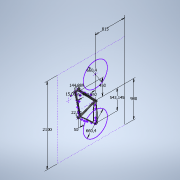
# Autodesk Inventor part: marco_bicicleta
Saved by Autodesk Inventor 2021 (Build 250183000, 183)
## iProperties
Created: 2021-06-19
Part Number: marco_bicicleta
Material: Generic
Document SubType Name: Modeling
Designer: j2seb
Density: 1 g/cm^3
Appearance: Default
Author: j2seb
Autodesk Inventor part; units mm, degrees
ref_plane "YZ Plane" through (0, 0, 0) normal (1, 0, 0) x (0, 1, 0)
ref_plane "XZ Plane" through (0, 0, 0) normal (0, 1, 0) x (-1, 0, 0)
sketch "Sketch1" plane through (0, 0, 0) normal (1, 0, 0) x (0, 1, 0)
  line L0 (-188.557163, 463.591927) -> (-1.253866, 0) construction
  line L1 (-1.253866, 0) -> (-1.253866, 463.591927) construction
  line L2 (-1.253866, 463.591927) -> (-188.557163, 463.591927) construction
  line L3 (-981.253866, 1020.526454) -> (1118.746134, 1020.526454) construction
  line L4 (1118.746134, 1020.526454) -> (1118.746134, -815) construction
  line L5 (1118.746134, -815) -> (-981.253866, -815) construction
  line L6 (-981.253866, -815) -> (-981.253866, 1020.526454) construction
  line L7 (-1.253866, 0) -> (-188.557163, 463.591927) construction
  spline S0 degree 4 poles (-1.253866, 0) (194.04307, 27.090506) (323.794867, 322.918039) (382.247207, 368.910907) (498.041645, 473.702936) knots 0 0 0 0 0 1 1 1 1 1 construction
  spline S1 degree 4 poles (412, 392) (351.287654, 407.817477) (266.833274, 424.891932) (92.672416, 474.286561) (-63.023498, 459.392893) (-169.985468, 435.393007) (-274.699695, 377.873475) (-355.05357, 267.227582) (-419.041856, 183.619141) (-523.324107, 44.784314) (-544.398866, 0) knots 0 0 0 0 0 0.24987965 0.35395029 0.45612478 0.55197991 0.64522658 0.74275576 1 1 1 1 1 construction
  spline S2 degree 4 poles (479.285201, 543.702936) (451.450857, 528.970628) (249.224988, 507.620964) (44.691003, 487.899446) (-77.02649, 451.650815) (-181.273608, 445.564496) knots 0 0 0 0 0 0.47207025 1 1 1 1 1 construction
  spline S3 degree 4 poles (-544.398866, 0) (-454.774301, 0) (-531.823407, 0) (-29.704647, 0) (-138.789942, 0) (-1.253866, 0) knots 0 0 0 0 0 0.47354405 1 1 1 1 1 construction
  line L8 (510.551387, 427.015943) -> (471.72853, 571.904817)
  line L9 (510.551387, 427.015943) -> (510.551387, 571.904817) construction
  line L10 (510.551387, 571.904817) -> (471.72853, 571.904817) construction
  circle A0 centre (-544.398866, 0) radius 330.2
  circle A1 centre (624.969964, 0) radius 330.2
  line L11 (-188.557163, 463.591927) -> (-1.253866, 0)
  line L12 (-1.253866, 0) -> (498.041645, 473.702936)
  line L13 (-544.398866, 0) -> (-1.253866, 0) construction
  line L14 (479.285201, 543.702936) -> (-168.355851, 413.591927)
  line L15 (-168.355851, 413.591927) -> (-544.398866, 0) construction
  point P0 (192.432816, 122.105258)
  point P1 (325.864172, 288.41297)
  point P2 (-173.723246, 426.876695)
  point P3 (322.192493, 413.760456)
  point P4 (197.332529, 441.76245)
  point P5 (49.344834, 462.975043)
  point P6 (-67.947241, 455.471589)
  point P7 (-268.511497, 370.782523)
  point P8 (-328.806584, 303.532756)
  point P9 (-385.39981, 227.949416)
  point P10 (-475.616953, 106.097259)
  point P11 (416.838074, 528.205777)
  point P12 (254.097905, 507.770061)
  point P13 (87.143519, 485.794364)
  point P14 (-40, 463.591927)
  point P15 (-409.001418, 0)
  point P16 (-196.045421, 0)
  point P17 (-112.874805, 0)
  point P18 (448.746134, 657.676287)
  point P19 (369.957321, 724.3169)
  point P20 (-473.317899, 0)
  dimension "d26" = 463.59193
  dimension "d27" = 22
  dimension "d28" = 15
  dimension "d29" = 144.88887
  dimension "d30" = 543.145
  dimension "d31" = 450
  dimension "d32" = 660.4
  dimension "d33" = 660.4
  dimension "d34" = 980
  dimension "d35" = 2100
  dimension "d36" = 815
  dimension "d37" = 70
  dimension "d72" = 50
  constraints: 24 end point, 8 point on line, 6 horizontal alignment, 5 coincident, 3 horizontal, 2 centre point, 2 vertical, 1 collinear, 1 perpendicular, 29 other
  measures "d26" vertical distance of L2.end L1.start
  measures "d27" angle of L1 L0
  measures "d28" angle of L8 L9
  measures "d29" distance of L9.start L9.end
  measures "d30" distance of L1.start point (-544.399, 0)
  measures "d31" horizontal distance of L1.start point (448.746, 657.676)
  measures "d32" diameter of A0
  measures "d33" diameter of A1
  measures "d34" horizontal distance of L5.end L1.start
  measures "d35" distance of L4.start L3.start
  measures "d36" vertical distance of L5.end L1.start
  measures "d37" vertical distance of L12.end L14.start
  measures "d72" vertical distance of L14.end L2.end
ref_plane "Work Plane1" through (0, 510.551387, 427.015943) normal (0, -0.258819, 0.9659258) x (1, 0, 0)
sketch "Sketch2" plane through (0, 510.551387, 427.015943) normal (0, -0.258819, 0.9659258) x (1, 0, 0)
  circle A0 centre (0, 0) radius 20
  circle A1 centre (0, 0) radius 17.5
  point P0 (0, -603.674629)
  dimension "d49" = 40
  dimension "d50" = 35
  constraints: 2 centre point, 1 coincident
  measures "d49" diameter of A0
  measures "d50" diameter of A1
extrude "Extrusion1" add sketch "Sketch2" along normal up to surface (150 mm away)
ref_plane "Work Plane3" through (0, -1.253866, 0) normal (0, 0.7254548, 0.6882699) x (-1, 0, 0)
sketch "Sketch3" plane through (0, -1.253866, 0) normal (0, 0.7254548, 0.6882699) x (-1, 0, 0)
  circle A0 centre (0, 0) radius 25
  circle A1 centre (0, 0) radius 22.5
  point P0 (0, -0.862998)
  dimension "d53" = 50
  dimension "d54" = 45
  constraints: 2 centre point, 1 coincident
  measures "d53" diameter of A0
  measures "d54" diameter of A1
extrude "Extrusion2" add sketch "Sketch3" along normal up to surface (688.251755 mm away) separate body
ref_plane "Work Plane4" through (0, -1.253866, 0) normal (0, 0.3746066, -0.9271839) x (-1, 0, 0)
sketch "Sketch4" plane through (0, -1.253866, 0) normal (0, 0.3746066, -0.9271839) x (-1, 0, 0)
  circle A0 centre (0, 0) radius 20
  circle A1 centre (0, 0) radius 17.5
  point P0 (0, 1.162564)
  dimension "d57" = 40
  dimension "d58" = 35
  constraints: 2 centre point, 1 coincident
  measures "d57" diameter of A0
  measures "d58" diameter of A1
extrude "Extrusion3" add sketch "Sketch4" against normal up to surface (500 mm away) separate body
ref_plane "Work Plane5" through (0, 479.285201, 543.702936) normal (0, -0.9804106, -0.1969644) x (1, 0, 0)
sketch "Sketch5" plane through (0, 479.285201, 543.702936) normal (0, -0.9804106, -0.1969644) x (1, 0, 0)
  circle A0 centre (0, 0) radius 20
  circle A1 centre (0, 0) radius 17.5
  point P0 (0, -438.650034)
  dimension "d73" = 40
  dimension "d74" = 35
  constraints: 2 centre point, 1 coincident
  measures "d73" diameter of A0
  measures "d74" diameter of A1
extrude "Extrusion4" add sketch "Sketch5" along normal up to surface (660.581417 mm away) separate body
ref_plane "Work Plane6" through (0, -168.355851, 413.591927) normal (0, 0.7398952, -0.6727221) x (1, 0, 0)
sketch "Sketch6" plane through (0, -168.355851, 413.591927) normal (0, 0.7398952, -0.6727221) x (1, 0, 0)
  line L0 (0, 0) -> (-47.280387, 244.90025)
  line L1 (-50, 273.334168) -> (-50, 558.987148)
  line L2 (-20, 193.601496) -> (-20, -23.404893)
  line L3 (0, 228.787148) -> (0, 889.187148) construction
  line L4 (0, 558.987148) -> (-50, 558.987148) construction
  arc A0 (-50, 273.334168) -> (-47.280387, 244.90025) centre (100, 273.334168) ccw
  point P0 (0, 192.757992)
  point P1 (-50, 258.987148)
  dimension "d77" = 50
  dimension "d78" = 300
  dimension "d79" = 150
  constraints: 6 end point, 2 point on circle, 2 point on line, 2 tangent, 1 centre point, 1 coincident, 1 horizontal, 1 parallel
  measures "d77" distance from line of L0.start L1
  measures "d78" distance of point (-50, 258.987) L1.end
  measures "d79" radius of A0
ref_plane "Work Plane7" through (-50, -544.398866, 0) normal (0, -0.6727221, -0.7398952) x (1, 0, 0)
sketch "Sketch7" plane through (-50, -544.398866, 0) normal (0, -0.6727221, -0.7398952) x (1, 0, 0)
  circle A0 centre (0, 0) radius 10
  circle A1 centre (0, 0) radius 7.5
  point P0 (50, -402.798127)
  dimension "d80" = 20
  dimension "d81" = 15
  constraints: 2 centre point, 1 coincident
  measures "d80" diameter of A0
  measures "d81" diameter of A1
sweep "Sweep1" add profiles "Sketch7" path "Sketch6" separate body path curves L1 A0 L0
mirror "Mirror1" about plane through (0, 0, 0) normal (1, 0, 0) bodies 5 separate body
sketch "Sketch8" plane through (0, 0, 0) normal (1, 0, 0) x (0, 1, 0)
  line L0 (15.95288, -18.136369) -> (-18.460612, 18.136369)
  circle A0 centre (-1.253866, 0) radius 25
  circle A1 centre (-1.253866, 0) radius 22.5
  point P0 (0, 0)
  dimension "d84" = 50
  dimension "d85" = 45
  constraints: 2 centre point, 1 coincident, 1 midpoint
  measures "d84" diameter of A0
  measures "d85" diameter of A1
extrude "Extrusion5" add sketch "Sketch8" along normal mid plane 72 separate body contours A0 L0 A1 | L0 A1 A0
ref_plane "Work Plane8" through (0, -473.317899, 0) normal (0, 0, 1) x (1, 0, 0)
sketch "Sketch9" plane through (0, -473.317899, 0) normal (0, 0, 1) x (1, 0, 0)
  ellipse E0 centre (0, 472.064033) end of major axis (-20, 472.064033) minor radius 18.543677
  ellipse E1 centre (-50, -71.080967) end of major axis (-40, -71.080967) minor radius 7.398952
  line L0 (20, 472.064033) -> (-20, 472.064033) construction
  line L1 (-20, 472.064033) -> (-49.613997, 235.119942)
  line L2 (-50, 228.919033) -> (-50, -71.080967)
  arc A0 (-49.613997, 235.119942) -> (-50, 228.919033) centre (0, 228.919033) ccw
  point P0 (0, 473.317899)
  dimension "d90" = 40
  dimension "d91" = 50
  dimension "d92" = 300
  constraints: 6 end point, 2 point on circle, 2 tangent, 1 centre point, 1 coincident, 1 horizontal, 1 midpoint, 1 vertical, 1 other
  measures "d90" distance of L0.start L0.end
  measures "d91" radius of A0
  measures "d92" distance of L2.start L2.end
ref_plane "Work Plane9" through (-50, -544.398866, 0) normal (0, -1, 0) x (1, 0, 0)
sketch "Sketch10" plane through (-50, -544.398866, 0) normal (0, -1, 0) x (1, 0, 0)
  circle A0 centre (0, 0) radius 10
  circle A1 centre (0, 0) radius 7.5
  point P0 (50, 0)
  dimension "d93" = 20
  dimension "d94" = 15
  constraints: 2 centre point, 1 coincident
  measures "d93" diameter of A0
  measures "d94" diameter of A1
sweep "Sweep2" add profiles "Sketch10" path "Sketch9" separate body path curves L2 A0 L1
mirror "Mirror2" about plane through (0, 0, 0) normal (1, 0, 0) bodies 8 separate body
sketch "Sketch11" plane through (36, -1.253866, 0) normal (1, 0, 0) x (0, 0, -1)
  circle A0 centre (0, 0) radius 25 projected
  point P0 (0, 1.253866)
extrude "Extrusion6" cut sketch "Sketch11" against normal blind 75 bodies 9 8 3 2
ref_plane "Work Plane10" through (0, 49.527967, 48.17889) normal (0, 0.7254548, 0.6882699) x (-1, 0, 0)
sketch "Sketch16" plane through (50, -544.398866, 0) normal (0, -1, 0) x (1, 0, 0)
  circle A0 centre (0, 0) radius 7.5 projected
  circle A1 centre (0, 0) radius 10 projected
  point P0 (-50, 0)
extrude "Extrusion8" cut sketch "Sketch16" against normal blind 30 bodies 9
sketch "Sketch17" plane through (-50, -544.398866, 0) normal (0, -1, 0) x (1, 0, 0)
  circle A0 centre (0, 0) radius 7.5 projected
  circle A1 centre (0, 0) radius 10 projected
  point P0 (50, 0)
extrude "Extrusion9" cut sketch "Sketch17" against normal blind 30 bodies 8
sketch "Sketch18" plane through (50, -544.398866, 0) normal (0, -0.6727221, -0.7398952) x (-1, 0, 0)
  circle A0 centre (0, 0) radius 7.5 projected
  circle A1 centre (0, 0) radius 10 projected
  point P0 (50, 402.798127)
extrude "Extrusion10" cut sketch "Sketch18" against normal blind 30 contours A0 | A1 bodies 6
sketch "Sketch19" plane through (-50, -544.398866, 0) normal (0, -0.6727221, -0.7398952) x (-1, 0, 0)
  circle A0 centre (0, 0) radius 10 projected
  point P0 (-50, 402.798127)
extrude "Extrusion11" cut sketch "Sketch19" against normal blind 30 bodies 5
sketch "Sketch20" plane through (0, -188.557163, 463.591927) normal (0, -0.3746066, 0.9271839) x (1, 0, 0)
  circle A0 centre (0, 0) radius 17.5
  circle A1 centre (0, 0) radius 20
  ellipse E0 centre (0, 0) end of major axis (-24.561532, -24.561532) minor radius 6.592592 (0, -9.159814) -> (0, 9.159814) ccw construction
  line L0 (0, 0) -> (0, -20) construction
  circle A2 centre (0, 0) radius 20 construction
  line L1 (-2.5, -15) -> (2.5, -15)
  line L2 (2.5, -15) -> (2.5, -20)
  line L3 (2.5, -20) -> (-2.5, -20)
  line L4 (-2.5, -20) -> (-2.5, -15)
  point P0 (0, 1.162564)
  point P1 (-2.5, -17.320508)
  point P2 (-2.5, -19.843135)
  point P3 (2.5, -19.843135)
  point P4 (2.5, -17.320508)
  dimension "d117" = 5
  dimension "d118" = 5
  constraints: 10 end point, 2 parallel, 1 horizontal, 1 midpoint, 1 perpendicular, 1 vertical, 1 vertical alignment, 2 other
  measures "d117" distance of L1.start L1.end
  measures "d118" distance between parallel lines of L3 L1
extrude "Extrusion12" cut sketch "Sketch20" against normal blind 23.975 contours A0 L2 A1 L4 picked at (0, -18.320017) bodies 3
sketch "Sketch21" plane through (0, -188.557163, 463.591927) normal (0, -0.3746066, 0.9271839) x (1, 0, 0)
  arc A0 (2.5, -17.320508) -> (-2.5, -17.320508) centre (0, 0) ccw
  arc A1 (2.5, -19.843135) -> (-2.5, -19.843135) centre (0, 0) ccw
  circle A2 centre (0, 0) radius 20
  point P0 (0, 1.162564)
  point P1 (-2.5, -19.843135)
  point P2 (2.5, -19.843135)
  constraints: 1 centre point, 1 coincident, 1 concentric
extrude "Extrusion13" cut sketch "Sketch21" against normal blind 566.9 bodies 4 6 5 7
sketch "Sketch22" plane through (0, 471.72853, 571.904817) normal (0, -0.258819, 0.9659258) x (1, 0, 0)
  circle A0 centre (0, 0) radius 20 projected
  point P0 (0, -603.674629)
extrude "Extrusion14" cut sketch "Sketch22" against normal up to surface (150 mm away) bodies 4 2
body "Solid1"
body "Solid2"
body "Solid3"
body "Solid4"
body "Solid5"
body "Solid6"
body "Solid7"
body "Solid8"
body "Solid9"
